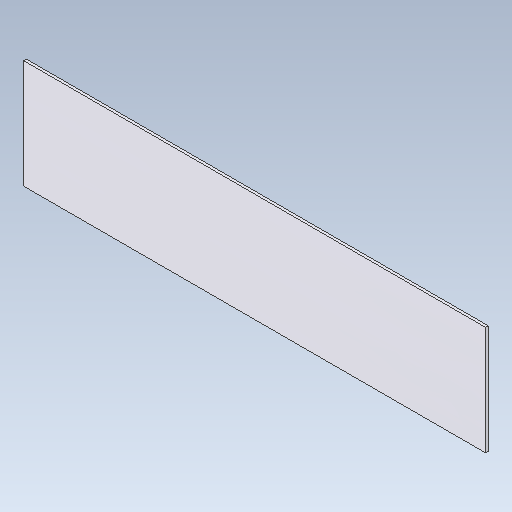
# Autodesk Inventor part: text
Saved by Autodesk Inventor 2020 (Build 240168000, 168)
## iProperties
Created: 2017-11-22
Part Number: text
Material: Generic
Document SubType Name: Modeling
Designer: stedrock
Density: 1 g/cm^3
Appearance: Default
Mass: 6.8 g
Surface Area: 140.2 cm^2
Volume: 6.8 cm^3
Author: stedrock
Autodesk Inventor part; units mm, degrees
ref_plane "YZ Plane" through (0, 0, 0) normal (1, 0, 0) x (0, 1, 0)
ref_plane "XZ Plane" through (0, 0, 0) normal (0, 1, 0) x (-1, 0, 0)
ref_plane "XY Plane" through (0, 0, 0) normal (0, 0, 1) x (1, 0, 0)
sketch "Sketch1" plane through (0, 0, 0) normal (0, 0, 1) x (1, 0, 0)
  line L0 (-85, -20) -> (85, -20)
  line L1 (85, -20) -> (85, 20)
  line L2 (85, 20) -> (-85, 20)
  line L3 (-85, 20) -> (-85, -20)
  line L4 (-85, -20) -> (85, 20) construction
  line L5 (85, -20) -> (-85, 20) construction
  line L6 (-72.8208, 17.2802) -> (71.9828, 17.2802) construction
  line L7 (71.9828, 17.2802) -> (71.9828, -17.2001) construction
  line L8 (71.9828, -17.2001) -> (-72.8208, -17.2001) construction
  line L9 (-72.8208, -17.2001) -> (-72.8208, 17.2802) construction
  point P0 (0, 0)
  dimension "d0" = 170
  dimension "d1" = 40
  constraints: 12 end point, 2 midpoint, 2 parallel, 1 horizontal, 1 perpendicular, 2 other
  measures "d0" distance of L2.end L1.end
  measures "d1" distance of L1.end L0.end
extrude "Extrusion1" add sketch "Sketch1" along normal blind 1
sketch "Sketch2" plane through (0, 0, 0) normal (0, 0, -1) x (-1, 0, 0)
  line L0 (-77.0434, 16.9651) -> (77.1762, 16.9651) construction
  line L1 (77.1762, 16.9651) -> (77.1762, -17.4121) construction
  line L2 (77.1762, -17.4121) -> (-77.0434, -17.4121) construction
  line L3 (-77.0434, -17.4121) -> (-77.0434, 16.9651) construction
  point P0 (0, 0)
  constraints: 2 other
body "Solid1"
